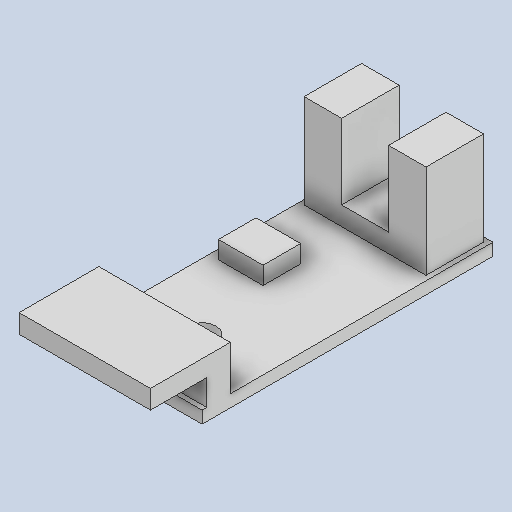
# Autodesk Inventor part: LM393 encoder
Saved by Autodesk Inventor 2022 (Build 260153070, 153G)
## iProperties
Created: 2021-11-27
Part Number: LM393 encoder
Material: Generic
Document SubType Name: Modeling
Designer: a laptop
Density: 1 g/cm^3
Appearance: Default
Author: a laptop
Autodesk Inventor part; units mm, degrees
ref_plane "YZ Plane" through (0, 0, 0) normal (1, 0, 0) x (0, 1, 0)
ref_plane "XZ Plane" through (0, 0, 0) normal (0, 1, 0) x (-1, 0, 0)
ref_plane "XY Plane" through (0, 0, 0) normal (0, 0, 1) x (1, 0, 0)
sketch "Sketch1" plane through (0, 0, 0) normal (0, 1, 0) x (-1, 0, 0)
  line L0 (0, -31) -> (14, -31)
  line L1 (14, -31) -> (14, 0)
  line L2 (14, 0) -> (7, 0)
  line L3 (0, 0) -> (0, -31)
  line L4 (0.5, -30.5) -> (13.5, -30.5)
  line L5 (13.5, -30.5) -> (13.5, -24.375)
  line L6 (13.5, -24.375) -> (0.5, -24.375)
  line L7 (0.5, -24.375) -> (0.5, -30.5)
  circle A0 centre (7, -7) radius 1.5
  line L8 (7, 0) -> (7, -31) construction
  line L9 (7, 0) -> (0, 0)
  line L10 (13, -14.75) -> (8.25, -14.75)
  line L11 (8.25, -14.75) -> (8.25, -18.75)
  line L12 (8.25, -18.75) -> (13, -18.75)
  line L13 (13, -18.75) -> (13, -14.75)
  dimension "d0" = 14
  dimension "d1" = 31
  dimension "d2" = 0.5
  dimension "d3" = 13
  dimension "d4" = 6.125
  dimension "d5" = 0.5
  dimension "d7" = 3
  dimension "d8" = 7
  dimension "d9" = 1
  dimension "d10" = 14.75
  dimension "d11" = 4
  dimension "d12" = 4.75
  constraints: 28 end point, 7 parallel, 3 horizontal, 3 perpendicular, 1 centre point, 1 coincident, 1 collinear, 1 midpoint, 1 point on line
  measures "d0" distance of L0.start L0.end
  measures "d1" distance of L0.end L1.end
  measures "d2" distance between parallel lines of L0 L4
  measures "d3" distance of L5.end L6.end
  measures "d4" distance of L6.end L4.start
  measures "d5" distance between parallel lines of L3 L7
  measures "d7" diameter of A0
  measures "d8" horizontal distance of L1.end A0.centre
  measures "d9" distance between parallel lines of L1 L13
  measures "d10" distance between parallel lines of L2 L10
  measures "d11" distance of L12.end L10.start
  measures "d12" distance of L10.start L10.end
extrude "Extrusion1" add sketch "Sketch1" against normal blind 1.3 contours L3 L9 L2 L1 L0 | L7 L6 L5 L4 | L13 L12 L11 L10
extrude "Extrusion2" add sketch "Sketch1" along normal blind 2 contours L7 L6 L5 L4
extrude "Extrusion3" add sketch "Sketch1" along normal blind 1.875 contours L13 L12 L11 L10
sketch "Sketch2" plane through (0, 2, 0) normal (0, 1, 0) x (1, 0, 0)
  line L0 (-13.5, 30.5) -> (-0.5, 30.5) projected
  line L1 (-0.5, 24.375) -> (-13.5, 24.375) projected
  line L2 (-4.5, 30.5) -> (-0.5, 30.5)
  line L3 (-0.5, 30.5) -> (-0.5, 24.375)
  line L4 (-0.5, 24.375) -> (-4.5, 24.375)
  line L5 (-4.5, 24.375) -> (-4.5, 30.5)
  line L6 (-13.5, 24.375) -> (-13.5, 30.5) projected
  line L7 (-13.5, 30.5) -> (-9.5, 30.5)
  line L8 (-9.5, 30.5) -> (-9.5, 24.375)
  line L9 (-9.5, 24.375) -> (-13.5, 24.375)
  line L10 (-13.5, 24.375) -> (-13.5, 30.5)
  point P0 (0, 0)
  dimension "d19" = 4
  dimension "d20" = 4
  constraints: 16 end point, 4 parallel, 2 horizontal, 2 perpendicular, 2 point on line
  measures "d19" distance between parallel lines of L3 L5
  measures "d20" distance between parallel lines of L6 L8
extrude "Extrusion4" add sketch "Sketch2" along normal blind 8 contours L0 L8 L1 L6 | L0 L3 L1 L5
sketch "Sketch3" plane through (0, 0, 0) normal (1, 0, 0) x (0, 1, 0)
  line L0 (0, 0) -> (0, -31) projected
  line L1 (0, -3) -> (4.75, -3)
  line L2 (4.75, -3) -> (4.75, -0.5)
  line L3 (4.75, -0.5) -> (0, -0.5)
  line L4 (0, -0.5) -> (0, -3)
  line L5 (0, 0) -> (-1.3, 0) projected
  line L6 (4.75, -0.5) -> (2.75, -0.5)
  line L7 (2.75, -0.5) -> (2.75, 5.5)
  line L8 (2.75, 5.5) -> (4.75, 5.5)
  line L9 (4.75, 5.5) -> (4.75, -0.5)
  point P0 (0, -0.5)
  dimension "d23" = 4.75
  dimension "d24" = 2.5
  dimension "d25" = 0.5
  dimension "d26" = 8.5
  dimension "d27" = 2
  constraints: 16 end point, 4 parallel, 2 horizontal, 2 perpendicular, 1 point on line
  measures "d23" distance of L1.start L1.end
  measures "d24" distance of L1.end L2.end
  measures "d25" distance between parallel lines of L5 L3
  measures "d26" distance of L8.end L1.end
  measures "d27" distance of L7.end L8.end
extrude "Extrusion5" add sketch "Sketch3" against normal up to surface (14 mm away)
body "Solid1"
